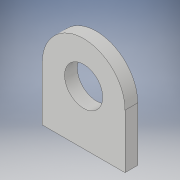
# Autodesk Inventor part: podporka_mala
Saved by Autodesk Inventor 2019 (Build 230136000, 136)
## iProperties
Created: 2019-12-14
Part Number: podporka_mala
Material: Ogólny
Document SubType Name: Modeling
Designer: Karolina
Density: 1 g/cm^3
Appearance: Domyślna
Author: Karolina
Autodesk Inventor part; units mm, degrees
ref_plane "YZ Plane" through (0, 0, 0) normal (1, 0, 0) x (0, 1, 0)
ref_plane "XZ Plane" through (0, 0, 0) normal (0, 1, 0) x (-1, 0, 0)
ref_plane "XY Plane" through (0, 0, 0) normal (0, 0, 1) x (1, 0, 0)
sketch "Szkic1" plane through (0, 0, 0) normal (0, 0, 1) x (1, 0, 0)
  line L0 (0, 0) -> (6.5, 0)
  line L1 (6.5, 0) -> (6.5, 7.5)
  line L2 (6.5, 7.5) -> (0, 7.5)
  line L3 (0, 7.5) -> (0, 0)
  point P0 (3.25, 4.25)
  dimension "d0" = 6.5
  dimension "d5" = 3.25
  dimension "d6" = 4.25
  constraints: 8 end point, 2 parallel, 1 horizontal, 1 perpendicular
  measures "d0" distance of L1.end L2.end
  measures "d5" distance from line of L2 point (3.25, 4.25)
  measures "d6" distance from line of L0 point (3.25, 4.25)
extrude "Wyciągnięcie proste1" add sketch "Szkic1" along normal mid plane 1
fillet "Zaokrąglenie1" radius 3.25 2 edges at (6.5, 7.5, 0) (0, 7.5, 0)
hole "Otwór1" at (3.25, 4.25, 0) direction (0, 0, -1) diameter 3 end through all both
